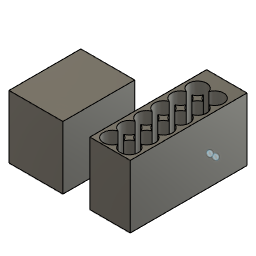
Sem+título (Autodesk Fusion 360 design; units mm, degrees)
Autodesk Fusion 360 part; units mm, degrees
sketch "Esboço1" plane through (0, 0, 0) normal (0, 1, 0) x (1, 0, 0)
  line L0 (0, 0) -> (-45, 0)
  line L1 (-45, 0) -> (-45, 130)
  line L2 (-45, 130) -> (0, 130)
  line L3 (0, 130) -> (0, 0)
  line L4 (-75, 0) -> (-135, 0)
  line L5 (-135, 0) -> (-135, 80)
  line L6 (-135, 80) -> (-75, 80)
  line L7 (-75, 80) -> (-75, 0)
  dimension "d1" = 45
  dimension "d2" = 130
  dimension "d3" = 60
  dimension "d4" = 80
  constraint horizontal L0
  constraint vertical L1
  constraint horizontal L2
  constraint vertical L3
  constraint coincident L0.start L3.end
  constraint horizontal L4
  constraint vertical L5
  constraint horizontal L6
  constraint vertical L7
  measures "d1" distance of L0.start L0.end
  measures "d2" distance of L0.start L2.end
  measures "d3" distance of L4.start L4.end
  measures "d4" distance of L4.start L6.end
extrude "Extrusão1" add sketch "Esboço1" along normal blind 70 makes body 1 at (-135, 23.3333, -26.6667) makes body 2 at (-45, 46.6667, -43.3333)
sketch "Esboço2" plane through (0, 70, 0) normal (0, 1, 0) x (-1, 0, 0)
  line L0 (0, -130) -> (45, -130)
  line L1 (45, -130) -> (45, 0)
  line L2 (45, 0) -> (0, 0)
  line L3 (0, 0) -> (0, -130)
  circle A0 centre (32, -12) radius 10
  circle A1 centre (13, -12) radius 10
  circle A2 centre (13, -31) radius 10
  circle A3 centre (32, -31) radius 10
  circle A4 centre (13, -50) radius 10
  circle A5 centre (32, -50) radius 10
  circle A6 centre (13, -69) radius 10
  circle A7 centre (32, -69) radius 10
  circle A8 centre (13, -88) radius 10
  circle A9 centre (32, -88) radius 10
  circle A10 centre (13, -107) radius 10
  circle A11 centre (32, -107) radius 10
  point P0 (32, -12)
  dimension "d7" = 20
  dimension "d8" = 20
  dimension "d9" = 20
  dimension "d10" = 20
  dimension "d11" = 20
  dimension "d12" = 20
  dimension "d13" = 20
  dimension "d14" = 20
  dimension "d15" = 20
  dimension "d16" = 20
  dimension "d17" = 20
  dimension "d18" = 20
  dimension "d21" = 13
  dimension "d22" = 13
  dimension "d23" = 19
  measures "d7" diameter of A0
  measures "d8" diameter of A1
  measures "d9" diameter of A3
  measures "d10" diameter of A2
  measures "d11" diameter of A5
  measures "d12" diameter of A4
  measures "d13" diameter of A7
  measures "d14" diameter of A6
  measures "d15" diameter of A9
  measures "d16" diameter of A8
  measures "d17" diameter of A11
  measures "d18" diameter of A10
  measures "d21" distance of L3 A1.centre
  measures "d22" distance of L1 P0
  measures "d23" distance of P0 A1.centre
extrude "Extrusão2" cut sketch "Esboço2" against normal blind 60 contours A0 A1 A3 | A0 A1 | A0 A1 A2 | A0 A2 A3 A5 | A0 A3 | A1 A2 | A1 A2 A3 A4 | A2 A4 | A2 A4 A5 A6 | A2 A3 | A3 A4 A5 A7 | A3 A5 | A4 A6 | A4 A6 A7 A8 | A4 A5 | A6 A8 | A6 A8 A9 A10 | A5 A6 A7 A9 | A5 A7 | A6 A7 | A8 A10 | A8 A10 A11 | A7 A8 A9 A11 | A8 A9 | A10 A11 | A9 A10 A11 | A7 A9 | A9 A11 bodies 2
sketch "Esboço4" plane through (0, 0, -130) normal (0, 0, -1) x (-1, 0, 0)
  line L0 (0, 0) -> (45, 0)
  line L1 (45, 0) -> (45, 70)
  line L2 (45, 70) -> (0, 70)
  line L3 (0, 70) -> (0, 0)
  line L4 (14.75, 11) -> (27.75, 11)
  line L5 (27.75, 11) -> (31.25, 8)
  line L6 (14.75, 11) -> (14.75, 2)
  line L7 (14.75, 11) -> (14.75, 2)
  line L8 (27.75, 11) -> (31.25, 8)
  line L9 (27.75, 2) -> (31.25, 5)
  line L10 (27.75, 2) -> (31.25, 5)
  line L11 (14.75, 11) -> (27.75, 11)
  line L12 (31.25, 8) -> (31.25, 5)
  line L13 (14.75, 2) -> (27.75, 2)
  line L14 (31.25, 8) -> (31.25, 5)
  line L15 (14.75, 2) -> (27.75, 2)
  line L16 (27.0102, 4) -> (29.25, 5.9199)
  line L17 (29.25, 7.0801) -> (29.25, 5.9199)
  line L18 (27.0102, 9) -> (29.25, 7.0801)
  line L19 (16.75, 9) -> (27.0102, 9)
  line L20 (16.75, 9) -> (16.75, 4)
  line L21 (16.75, 4) -> (27.0102, 4)
  dimension "d25" = 9
  dimension "d26" = 16.5
  dimension "d27" = 13
  dimension "d28" = 13
  dimension "d29" = 3
  dimension "d30" = 9
  dimension "d31" = 2
  measures "d25" distance of L4 L13
  measures "d26" distance of L6 L12
  measures "d27" distance of L4.start L4.end
  measures "d28" distance of L9.start L6.end
  measures "d29" distance of L5.end L9.end
  measures "d30" distance of L4.start L6.end
extrude "Extrusão3" cut sketch "Esboço4" against normal blind 7.7 contours L4 L5 L6 L7 L8 L9 L10 L11 L12 L13 L14 L15 bodies 2
extrude "Extrusão4" cut 1 faces at (-20.1701, 7.3333, -130) along direction (0, 0, 1) blind 15.5 on bodies 2 bodies 2
sketch "Esboço5" plane through (0, 0, -114.5) normal (0, 0, -1) x (-1, 0, 0)
  line L0 (27.0102, 9) -> (16.75, 9)
  line L1 (16.75, 9) -> (16.75, 4)
  line L2 (16.75, 4) -> (27.0102, 4)
  line L3 (27.0102, 4) -> (29.25, 5.9199)
  line L4 (29.25, 5.9199) -> (29.25, 7.0801)
  line L5 (29.25, 7.0801) -> (27.0102, 9)
  circle A0 centre (19.3225, 6.5) radius 2.5063
  circle A1 centre (25.7906, 6.5) radius 2.5022
